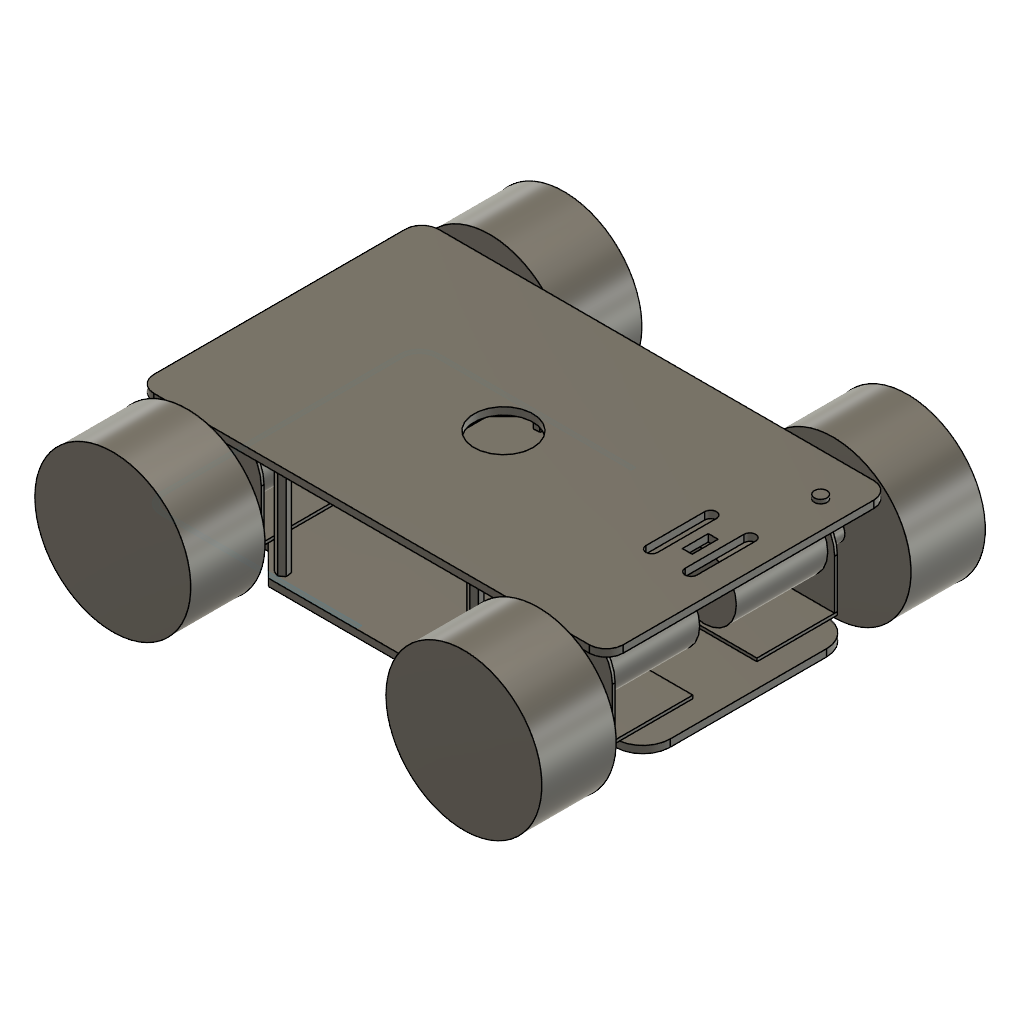
chassi migo base (Autodesk Fusion 360 design; units mm, degrees)
Autodesk Fusion 360 part; units mm, degrees
sketch "Esboço1" plane through (0, 0, 0) normal (0, 1, 0) x (1, 0, 0)
  line L0 (0, 0) -> (0, -111.6)
  line L1 (0, -111.6) -> (50, -111.6)
  line L2 (50, -111.6) -> (65.6125, -127.1)
  line L3 (65.6125, -127.1) -> (165.6125, -127.1)
  line L4 (165.6125, -127.1) -> (178.9919, -109.636)
  line L5 (178.9919, -109.636) -> (238.9919, -109.636)
  line L6 (238.9919, -109.636) -> (238.9919, -1.964)
  line L7 (238.9919, -1.964) -> (178.9919, -1.964)
  line L8 (178.9919, -1.964) -> (165.6125, 15.5)
  line L9 (165.6125, 15.5) -> (65.6125, 15.5)
  line L10 (65.6125, 15.5) -> (50, 0)
  line L11 (50, 0) -> (0, 0)
  dimension "d1" = 111.6
  dimension "d2" = 15.5
  dimension "d3" = 100
  dimension "d5" = 239
  dimension "d10" = 100
  dimension "d15" = 50
  dimension "d17" = 22
  dimension "d18" = 50
  dimension "d20" = 22
  dimension "d21" = 22
  dimension "d23" = 60
  dimension "d24" = 22
  dimension "d25" = 15.5
  dimension "d26" = 60
  constraint coincident L0.start L11.end
  constraint vertical L0
  constraint perpendicular L0 L1
  constraint perpendicular L0 L3
  constraint parallel L3 L5
  constraint perpendicular L5 L6
  constraint perpendicular L6 L7
  constraint perpendicular L6 L9
  constraint perpendicular L0 L11
  measures "d1" distance of L0.start L0.end
  measures "d2" distance of L1 L3
  measures "d3" distance of L2.end L3.end
  measures "d5" distance of L0.end L5.end
  measures "d10" distance of L8.end L9.end
  measures "d15" distance of L0.end L1.end
  measures "d17" distance of L1.end L2.end
  measures "d18" distance of L0.start L10.end
  measures "d20" distance of L7.end L8.end
  measures "d21" distance of L9.end L10.end
  measures "d23" distance of L6.end L7.end
  measures "d24" distance of L3.end L4.end
  measures "d25" vertical distance of L0.start L9.end
  measures "d26" distance of L4.end L5.end
extrude "Extrusão1" add sketch "Esboço1" along normal blind 3.7 makes body 1
fillet "Arredondamento1" radius 10 1 edges at (0, 1.85, 111.6) on bodies 1
fillet "Arredondamento2" radius 10 1 edges at (0, 1.85, 0) on bodies 1
fillet "Arredondamento3" radius 14 1 edges at (238.9919, 1.85, 109.636) on bodies 1
fillet "Arredondamento4" radius 14 1 edges at (238.9919, 1.85, 1.964) on bodies 1
sketch "Esboço2" plane through (0, 3.7, 0) normal (0, 1, 0) x (-1, 0, 0)
  arc A0 (-238.9919, 15.964) -> (-224.9919, 1.964) centre (-224.9919, 15.964) ccw
  line L0 (-224.9919, 1.964) -> (-178.9919, 1.964)
  line L1 (-178.9919, 1.964) -> (-165.6125, -15.5)
  line L2 (-165.6125, -15.5) -> (-65.6125, -15.5)
  line L3 (-65.6125, -15.5) -> (-50, 0)
  line L4 (-50, 0) -> (-10, 0)
  arc A1 (-10, 0) -> (0, 10) centre (-10, 10) ccw
  line L5 (0, 10) -> (0, 101.6)
  arc A2 (0, 101.6) -> (-10, 111.6) centre (-10, 101.6) ccw
  line L6 (-10, 111.6) -> (-50, 111.6)
  line L7 (-50, 111.6) -> (-65.6125, 127.1)
  line L8 (-65.6125, 127.1) -> (-165.6125, 127.1)
  line L9 (-165.6125, 127.1) -> (-178.9919, 109.636)
  line L10 (-178.9919, 109.636) -> (-224.9919, 109.636)
  arc A3 (-224.9919, 109.636) -> (-238.9919, 95.636) centre (-224.9919, 95.636) ccw
  line L11 (-238.9919, 95.636) -> (-238.9919, 15.964)
  line L12 (-69.4965, 121.884) -> (-69.0799, 118.7943)
  line L13 (-69.0799, 118.7943) -> (-66.1958, 117.6103)
  line L14 (-66.1958, 117.6103) -> (-63.7283, 119.516)
  line L15 (-63.7283, 119.516) -> (-64.145, 122.6057)
  line L16 (-64.145, 122.6057) -> (-67.0291, 123.7897)
  line L17 (-67.0291, 123.7897) -> (-69.4965, 121.884)
  line L18 (-167.5652, 122.0119) -> (-167.2872, 118.9067)
  line L19 (-167.2872, 118.9067) -> (-164.459, 117.5947)
  line L20 (-164.459, 117.5947) -> (-161.9087, 119.3881)
  line L21 (-161.9087, 119.3881) -> (-162.1867, 122.4933)
  line L22 (-162.1867, 122.4933) -> (-165.0149, 123.8053)
  line L23 (-165.0149, 123.8053) -> (-167.5652, 122.0119)
  line L24 (-70.3397, -6.4973) -> (-71.7356, -9.2851)
  line L25 (-71.7356, -9.2851) -> (-70.0192, -11.8878)
  line L26 (-70.0192, -11.8878) -> (-66.907, -11.7027)
  line L27 (-66.907, -11.7027) -> (-65.5112, -8.9149)
  line L28 (-65.5112, -8.9149) -> (-67.2275, -6.3122)
  line L29 (-67.2275, -6.3122) -> (-70.3397, -6.4973)
  line L30 (-167.9928, -8.5248) -> (-166.9588, -11.4661)
  line L31 (-166.9588, -11.4661) -> (-163.8946, -12.0412)
  line L32 (-163.8946, -12.0412) -> (-161.8644, -9.6752)
  line L33 (-161.8644, -9.6752) -> (-162.8984, -6.7339)
  line L34 (-162.8984, -6.7339) -> (-165.9625, -6.1588)
  line L35 (-165.9625, -6.1588) -> (-167.9928, -8.5248)
  point P0 (-66.6124, 120.7)
  point P1 (-164.7369, 120.7)
  point P2 (-68.6234, -9.1)
  point P3 (-164.9286, -9.1)
  dimension "d37" = 2.7
  dimension "d38" = 2.7
  dimension "d39" = 2.7
  dimension "d40" = 2.7
  dimension "d41" = 6.4
  dimension "d42" = 6.4
  dimension "d43" = 6.4
  dimension "d44" = 6.4
  measures "d37" distance of P0 L17
  measures "d38" distance of P1 L23
  measures "d39" distance of P2 L29
  measures "d40" distance of P3 L35
  measures "d41" distance of L8 P0
  measures "d42" distance of L8 P1
  measures "d43" distance of L2 P3
  measures "d44" distance of L2 P2
extrude "Extrusão2" add sketch "Esboço2" along normal blind 50 contours L12 L13 L14 L15 L16 L17 | L18 L19 L20 L21 L22 L23 | L24 L25 L26 L27 L28 L29 | L30 L31 L32 L33 L34 L35 bodies 1
sketch "Esboço3" plane through (0, 3.7, 0) normal (0, 1, 0) x (-1, 0, 0)
  line L0 (-67.2275, -6.3122) -> (-65.5112, -8.9149)
  line L1 (-65.5112, -8.9149) -> (-66.907, -11.7027)
  line L2 (-66.907, -11.7027) -> (-70.0192, -11.8878)
  line L3 (-70.0192, -11.8878) -> (-71.7356, -9.2851)
  line L4 (-71.7356, -9.2851) -> (-70.3397, -6.4973)
  line L5 (-70.3397, -6.4973) -> (-67.2275, -6.3122)
  line L6 (-67.0291, 123.7897) -> (-64.145, 122.6057)
  line L7 (-64.145, 122.6057) -> (-63.7283, 119.516)
  line L8 (-63.7283, 119.516) -> (-66.1958, 117.6103)
  line L9 (-66.1958, 117.6103) -> (-69.0799, 118.7943)
  line L10 (-69.0799, 118.7943) -> (-69.4965, 121.884)
  line L11 (-69.4965, 121.884) -> (-67.0291, 123.7897)
  line L12 (-165.9625, -6.1588) -> (-162.8984, -6.7339)
  line L13 (-162.8984, -6.7339) -> (-161.8644, -9.6752)
  line L14 (-161.8644, -9.6752) -> (-163.8946, -12.0412)
  line L15 (-163.8946, -12.0412) -> (-166.9588, -11.4661)
  line L16 (-166.9588, -11.4661) -> (-167.9928, -8.5248)
  line L17 (-167.9928, -8.5248) -> (-165.9625, -6.1588)
  line L18 (-165.0149, 123.8053) -> (-162.1867, 122.4933)
  line L19 (-162.1867, 122.4933) -> (-161.9087, 119.3881)
  line L20 (-161.9087, 119.3881) -> (-164.459, 117.5947)
  line L21 (-164.459, 117.5947) -> (-167.2872, 118.9067)
  line L22 (-167.2872, 118.9067) -> (-167.5652, 122.0119)
  line L23 (-167.5652, 122.0119) -> (-165.0149, 123.8053)
  arc A0 (-238.9919, 15.964) -> (-224.9919, 1.964) centre (-224.9919, 15.964) ccw
  line L24 (-224.9919, 1.964) -> (-178.9919, 1.964)
  line L25 (-178.9919, 1.964) -> (-165.6125, -15.5)
  line L26 (-165.6125, -15.5) -> (-65.6125, -15.5)
  line L27 (-65.6125, -15.5) -> (-50, 0)
  line L28 (-50, 0) -> (-10, 0)
  arc A1 (-10, 0) -> (0, 10) centre (-10, 10) ccw
  line L29 (0, 10) -> (0, 101.6)
  arc A2 (0, 101.6) -> (-10, 111.6) centre (-10, 101.6) ccw
  line L30 (-10, 111.6) -> (-50, 111.6)
  line L31 (-50, 111.6) -> (-65.6125, 127.1)
  line L32 (-65.6125, 127.1) -> (-165.6125, 127.1)
  line L33 (-165.6125, 127.1) -> (-178.9919, 109.636)
  line L34 (-178.9919, 109.636) -> (-224.9919, 109.636)
  arc A3 (-224.9919, 109.636) -> (-238.9919, 95.636) centre (-224.9919, 95.636) ccw
  line L35 (-238.9919, 95.636) -> (-238.9919, 15.964)
sketch "Esboço4" plane through (0, 3.7, 0) normal (0, 1, 0) x (-1, 0, 0)
  line L0 (-10, 74.1) -> (-50, 74.1)
  line L1 (-50, 74.1) -> (-50, 115.1)
  line L2 (-50, 115.1) -> (-10, 115.1)
  line L3 (-10, 115.1) -> (-10, 74.1)
  line L4 (0, 10) -> (0, 101.6)
  line L5 (-10, 111.6) -> (-50, 111.6)
  dimension "d47" = 10
  dimension "d48" = 40
  dimension "d49" = 41
  dimension "d50" = 3.5
  constraint horizontal L0
  constraint vertical L1
  constraint horizontal L2
  constraint vertical L3
  measures "d47" distance of L3 L4
  measures "d48" distance of L1.end L2.end
  measures "d49" distance of L0.end L1.end
  measures "d50" distance of L2 L5
sketch "Esboço5" plane through (0, 3.7, 0) normal (0, 1, 0) x (-1, 0, 0)
  line L0 (-186.9919, 72.136) -> (-226.9919, 72.136)
  line L1 (-226.9919, 72.136) -> (-226.9919, 113.136)
  line L2 (-226.9919, 113.136) -> (-186.9919, 113.136)
  line L3 (-186.9919, 113.136) -> (-186.9919, 72.136)
  line L4 (-238.9919, 95.636) -> (-238.9919, 15.964)
  line L5 (-178.9919, 109.636) -> (-224.9919, 109.636)
  dimension "d51" = 12
  dimension "d52" = 40
  dimension "d53" = 41
  dimension "d54" = 3.5
  constraint horizontal L0
  constraint vertical L1
  constraint horizontal L2
  constraint vertical L3
  measures "d51" distance of L1 L4
  measures "d52" distance of L0.start L0.end
  measures "d53" distance of L0.start L2.end
  measures "d54" distance of L2 L5
sketch "Esboço6" plane through (0, 3.7, 0) normal (0, 1, 0) x (-1, 0, 0)
  line L0 (-10, -3.5) -> (-50, -3.5)
  line L1 (-50, -3.5) -> (-50, 37.5)
  line L2 (-50, 37.5) -> (-10, 37.5)
  line L3 (-10, 37.5) -> (-10, -3.5)
  line L4 (-186.9919, -1.536) -> (-226.9919, -1.536)
  line L5 (-226.9919, -1.536) -> (-226.9919, 39.464)
  line L6 (-226.9919, 39.464) -> (-186.9919, 39.464)
  line L7 (-186.9919, 39.464) -> (-186.9919, -1.536)
  line L8 (-238.9919, 95.636) -> (-238.9919, 15.964)
  line L9 (-224.9919, 1.964) -> (-178.9919, 1.964)
  line L10 (0, 10) -> (0, 101.6)
  line L11 (-50, 0) -> (-10, 0)
  dimension "d55" = 40
  dimension "d56" = 41
  dimension "d57" = 40
  dimension "d58" = 41
  dimension "d59" = 12
  dimension "d61" = 3.5
  dimension "d62" = 10
  dimension "d63" = 3.5
  constraint horizontal L0
  constraint vertical L1
  constraint horizontal L2
  constraint vertical L3
  constraint horizontal L4
  constraint vertical L5
  constraint horizontal L6
  constraint vertical L7
  measures "d55" distance of L0.start L0.end
  measures "d56" distance of L0.start L2.end
  measures "d57" distance of L4.start L4.end
  measures "d58" distance of L4.start L6.end
  measures "d59" distance of L5 L8
  measures "d61" distance of L4 L9
  measures "d62" distance of L3 L10
  measures "d63" distance of L0 L11
extrude "Extrusão3" add sketch "Esboço6" sketch "Esboço4" sketch "Esboço5" along normal blind 1.6 of sketch 2 of sketch 3 bodies 1
sketch "Esboço7" plane through (0, 5.3, 0) normal (0, 1, 0) x (-1, 0, 0)
  line L0 (-10, 115.1) -> (-50, 115.1)
  line L1 (-50, 115.1) -> (-50, 74.1)
  line L2 (-50, 74.1) -> (-10, 74.1)
  line L3 (-10, 74.1) -> (-10, 115.1)
  line L4 (-10, 113.7) -> (-10, 115.1)
  line L5 (-10, 115.1) -> (-50, 115.1)
  line L6 (-50, 115.1) -> (-50, 113.7)
  line L7 (-50, 113.7) -> (-10, 113.7)
  dimension "d66" = 1.4
  constraint coincident L3 L4.start
  constraint coincident L0.start L3.end
  constraint coincident L0.end L1.start
  constraint coincident L1 L6.end
  constraint perpendicular L3 L7
  measures "d66" distance of L4.start L0.start
extrude "Extrusão4" add sketch "Esboço7" along normal blind 45.2 contours L0 L1 L3 L4 L5 L6 L7 bodies 1
sketch "Esboço8" plane through (0, 3.7, 0) normal (0, 1, 0) x (-1, 0, 0)
  line L0 (-0.1486, -16.5845) -> (-239.1486, -16.5845)
  line L1 (-239.1486, -16.5845) -> (-239.1486, 128.4155)
  line L2 (-239.1486, 128.4155) -> (-0.1486, 128.4155)
  line L3 (-0.1486, 128.4155) -> (-0.1486, -16.5845)
  line L4 (-238.9919, 95.636) -> (-238.9919, 15.964)
  dimension "d69" = 239
  dimension "d70" = 145
  constraint horizontal L0
  constraint vertical L1
  constraint horizontal L2
  constraint vertical L3
  measures "d69" distance of L0.start L0.end
  measures "d70" distance of L0.start L2.end
extrude "Extrusão5" add sketch "Esboço8" along normal blind 3.7 from surface at 50 bodies 1
fillet "Arredondamento5" radius 8.6 1 edges at (239.1486, 55.55, -16.5845) on bodies 1
fillet "Arredondamento6" radius 8.6 1 edges at (239.1486, 55.55, 128.4155) on bodies 1
fillet "Arredondamento7" radius 8.4 1 edges at (0.1486, 55.55, -16.5845) on bodies 1
fillet "Arredondamento8" radius 8.4 1 edges at (0.1486, 55.55, 128.4155) on bodies 1
fillet "Arredondamento9" radius 20 1 edges at (10, 50.5, 114.4) on bodies 1
fillet "Arredondamento10" radius 20 1 edges at (50, 50.5, 114.4) on bodies 1
sketch "Esboço9" plane through (0, 0, 115.1) normal (0, 0, 1) x (1, 0, 0)
  arc A0 (50, 30.5) -> (10, 30.5) centre (30, 30.5) ccw
  line L0 (10, 30.5) -> (10, 3.7)
  line L1 (10, 3.7) -> (50, 3.7)
  line L2 (50, 3.7) -> (50, 30.5)
  circle A1 centre (30, 23.7) radius 5.9
  dimension "d87" = 20
  dimension "d88" = 11.8
  measures "d87" distance of L1 A1.centre
  measures "d88" diameter of A1
extrude "Extrusão6" add sketch "Esboço9" along normal blind 5.8 contours A1 bodies 1
sketch "Esboço10" plane through (0, 0, 120.9) normal (0, 0, 1) x (1, 0, 0)
  circle A0 centre (30, 23.7) radius 5.9
  circle A1 centre (30, 23.7) radius 2.9
  dimension "d91" = 5.8
  constraint concentric A0 A1
  measures "d91" diameter of A1
extrude "Extrusão7" add sketch "Esboço10" along normal blind 15.4 contours A1 bodies 1
sketch "Esboço11" plane through (0, 0, 113.7) normal (0, 0, -1) x (-1, 0, 0)
  arc A0 (-10, 30.5) -> (-50, 30.5) centre (-30, 30.5) ccw
  line L0 (-50, 30.5) -> (-50, 5.3)
  line L1 (-50, 5.3) -> (-10, 5.3)
  line L2 (-10, 5.3) -> (-10, 30.5)
  circle A1 centre (-30, 30.5) radius 16.5
  dimension "d94" = 33
  constraint coincident A0.centre A1.centre
  measures "d94" diameter of A1
extrude "Extrusão8" add sketch "Esboço11" along normal blind 46.6 contours A1 bodies 1
sketch "Esboço12" plane through (0, 0, 0) normal (0, 0, 1) x (1, 0, 0)
  line L0 (10, 5.3) -> (50, 5.3)
  line L1 (50, 5.3) -> (50, 30.5)
  arc A0 (50, 30.5) -> (10, 30.5) centre (30, 30.5) ccw
  line L2 (10, 30.5) -> (10, 5.3)
extrude "Extrusão9" add sketch "Esboço12" along normal blind 1.4 from surface at -3.5 bodies 1
sketch "Esboço13" plane through (0, 0, 0) normal (0, 0, 1) x (1, 0, 0)
  circle A0 centre (30, 30.5) radius 16.5
extrude "Extrusão10" add sketch "Esboço13" along normal blind 46.6 from surface at -2.1 bodies 1
sketch "Esboço14" plane through (0, 0, 0) normal (0, 0, 1) x (1, 0, 0)
  circle A0 centre (30, 23.7) radius 5.9
extrude "Extrusão11" add sketch "Esboço14" along normal blind 5.8 from surface at -9.3 bodies 1
sketch "Esboço15" plane through (0, 0, 0) normal (0, 0, 1) x (1, 0, 0)
  circle A0 centre (30, 23.7) radius 2.9
extrude "Extrusão12" add sketch "Esboço15" along normal blind 15.4 from surface at -24.7 bodies 1
sketch "Esboço16" plane through (0, 0, 0) normal (0, 0, 1) x (1, 0, 0)
  line L0 (186.99, 5.3) -> (226.99, 5.3)
  line L1 (226.99, 5.3) -> (226.99, 30.5)
  arc A0 (226.99, 30.5) -> (186.99, 30.5) centre (206.99, 30.5) ccw
  line L2 (186.99, 30.5) -> (186.99, 5.3)
extrude "Extrusão13" add sketch "Esboço16" along normal blind 1.4 from surface at -1.54 bodies 1
sketch "Esboço17" plane through (0, 0, 0) normal (0, 0, 1) x (1, 0, 0)
  circle A0 centre (206.99, 30.5) radius 16.5
extrude "Extrusão14" add sketch "Esboço17" along normal blind 46.6 from surface at -0.14 bodies 1
sketch "Esboço18" plane through (0, 0, 0) normal (0, 0, 1) x (1, 0, 0)
  circle A0 centre (206.99, 23.7) radius 5.9
extrude "Extrusão15" add sketch "Esboço18" along normal blind 5.8 from surface at -7.34 bodies 1
sketch "Esboço19" plane through (0, 0, 0) normal (0, 0, 1) x (1, 0, 0)
  circle A0 centre (206.99, 23.7) radius 2.9
extrude "Extrusão16" add sketch "Esboço19" along normal blind 15.4 from surface at -22.74 bodies 1
sketch "Esboço20" plane through (0, 0, 0) normal (0, 0, 1) x (1, 0, 0)
  line L0 (186.99, 5.3) -> (226.99, 5.3)
  line L1 (226.99, 5.3) -> (226.99, 30.5)
  arc A0 (226.99, 30.5) -> (186.99, 30.5) centre (206.99, 30.5) ccw
  line L2 (186.99, 30.5) -> (186.99, 5.3)
extrude "Extrusão17" add sketch "Esboço20" along normal blind 1.4 from surface at 111.74 bodies 1
sketch "Esboço21" plane through (0, 0, 0) normal (0, 0, 1) x (1, 0, 0)
  circle A0 centre (206.99, 30.5) radius 16.5
extrude "Extrusão18" add sketch "Esboço21" along normal blind 46.6 from surface at 65.14 bodies 1
sketch "Esboço22" plane through (0, 0, 0) normal (0, 0, 1) x (1, 0, 0)
  circle A0 centre (206.99, 23.7) radius 5.9
extrude "Extrusão19" add sketch "Esboço22" along normal blind 5.8 from surface at 113.14 bodies 1
sketch "Esboço23" plane through (0, 0, 0) normal (0, 0, 1) x (1, 0, 0)
  circle A0 centre (206.99, 23.7) radius 2.9
extrude "Extrusão20" add sketch "Esboço23" along normal blind 15.4 from surface at 118.94 bodies 1
sketch "Esboço24" plane through (0, 57.4, 0) normal (0, 1, 0) x (-1, 0, 0)
  arc A0 (-0.1486, 120.0155) -> (-8.5486, 128.4155) centre (-8.5486, 120.0155) ccw
  line L0 (-8.5486, 128.4155) -> (-230.5486, 128.4155)
  arc A1 (-230.5486, 128.4155) -> (-239.1486, 119.8155) centre (-230.5486, 119.8155) ccw
  line L1 (-239.1486, 119.8155) -> (-239.1486, -7.9845)
  arc A2 (-239.1486, -7.9845) -> (-230.5486, -16.5845) centre (-230.5486, -7.9845) ccw
  line L2 (-230.5486, -16.5845) -> (-8.5486, -16.5845)
  arc A3 (-8.5486, -16.5845) -> (-0.1486, -8.1845) centre (-8.5486, -8.1845) ccw
  line L3 (-0.1486, -8.1845) -> (-0.1486, 120.0155)
sketch "Esboço25" plane through (0, 57.4, 0) normal (0, 1, 0) x (-1, 0, 0)
  circle A0 centre (-225, 5) radius 3.2443
extrude "Extrusão21" add sketch "Esboço25" along normal blind 2 bodies 1
sketch "Esboço26" plane through (0, 57.4, 0) normal (0, 1, 0) x (-1, 0, 0)
  circle A0 centre (-114.1486, 55.8) radius 15
  line L0 (-239.1486, 119.8155) -> (-239.1486, -7.9845)
  line L1 (-8.5486, 128.4155) -> (-230.5486, 128.4155)
  line L2 (-65.6125, 127.1) -> (-165.6125, 127.1)
  dimension "d135" = 30
  dimension "d136" = 125
  dimension "d139" = 71.3
  measures "d135" diameter of A0
  measures "d136" distance of A0.centre L0
  measures "d139" distance of A0.centre L2
extrude "Extrusão22" cut sketch "Esboço26" against normal blind 4 bodies 1
sketch "Esboço27" plane through (0, 57.4, 0) normal (0, 1, 0) x (-1, 0, 0)
  line L0 (-227.1486, 73.2155) -> (-221.1486, 73.2155)
  line L1 (-221.1486, 73.2155) -> (-221.1486, 37.2155)
  line L2 (-221.1486, 37.2155) -> (-227.1486, 37.2155)
  line L3 (-227.1486, 37.2155) -> (-227.1486, 73.2155)
  line L4 (-207.1486, 73.2155) -> (-201.1486, 73.2155)
  line L5 (-201.1486, 73.2155) -> (-201.1486, 37.2155)
  line L6 (-201.1486, 37.2155) -> (-207.1486, 37.2155)
  line L7 (-207.1486, 37.2155) -> (-207.1486, 73.2155)
  line L8 (-216.7486, 62.2155) -> (-211.7486, 62.2155)
  line L9 (-211.7486, 62.2155) -> (-211.7486, 49.0155)
  line L10 (-211.7486, 49.0155) -> (-216.7486, 49.0155)
  line L11 (-216.7486, 49.0155) -> (-216.7486, 62.2155)
  line L12 (-239.1486, 119.8155) -> (-239.1486, -7.9845)
  line L13 (-8.5486, 128.4155) -> (-230.5486, 128.4155)
  dimension "d142" = 6
  dimension "d143" = 36
  dimension "d144" = 6
  dimension "d145" = 36
  dimension "d146" = 5
  dimension "d147" = 13.2
  dimension "d148" = 12
  dimension "d149" = 55.2
  dimension "d150" = 55.2
  dimension "d151" = 66.2
  dimension "d152" = 32
  dimension "d153" = 22.4
  constraint horizontal L0
  constraint vertical L1
  constraint horizontal L2
  constraint vertical L3
  constraint horizontal L4
  constraint vertical L5
  constraint horizontal L6
  constraint vertical L7
  constraint horizontal L8
  constraint vertical L9
  constraint horizontal L10
  constraint vertical L11
  measures "d142" distance of L0.start L0.end
  measures "d143" distance of L0.start L2.end
  measures "d144" distance of L4.start L4.end
  measures "d145" distance of L4.start L6.end
  measures "d146" distance of L8.start L8.end
  measures "d147" distance of L8.start L10.end
  measures "d148" distance of L3 L12
  measures "d149" distance of L0 L13
  measures "d150" distance of L4 L13
  measures "d151" distance of L8 L13
  measures "d152" distance of L7 L12
  measures "d153" distance of L11 L12
extrude "Extrusão23" cut sketch "Esboço27" against normal blind 4 bodies 1
fillet "Arredondamento11" radius 3 4 edges at (221.1486, 55.55, 73.2155) (227.1486, 55.55, 73.2155) (221.1486, 55.55, 37.2155) (227.1486, 55.55, 37.2155) on bodies 1
fillet "Arredondamento12" radius 3 4 edges at (207.1486, 55.55, 37.2155) (201.1486, 55.55, 37.2155) (201.1486, 55.55, 73.2155) (207.1486, 55.55, 73.2155) on bodies 1
sketch "Esboço28" plane through (0, 0, 0) normal (0, 0, 1) x (1, 0, 0)
  circle A0 centre (30, 23.7) radius 40
sketch "Esboço29" plane through (0, 0, 0) normal (0, 0, 1) x (1, 0, 0)
  circle A0 centre (206.99, 23.7) radius 40
sketch "Esboço30" plane through (0, 0, 0) normal (0, 0, 1) x (1, 0, 0)
  circle A0 centre (206.99, 23.7) radius 40
sketch "Esboço31" plane through (0, 0, 0) normal (0, 0, 1) x (1, 0, 0)
  circle A0 centre (30, 23.7) radius 40
sketch "Esboço32" plane through (0, 0, 0) normal (0, 0, 1) x (1, 0, 0)
  circle A0 centre (30, 23.7) radius 6
sketch "Esboço33" plane through (0, 0, 0) normal (0, 0, 1) x (1, 0, 0)
  circle A0 centre (30, 23.7) radius 39.75
sketch "Esboço34" plane through (0, 0, 0) normal (0, 0, 1) x (1, 0, 0)
  circle A0 centre (206.99, 23.7) radius 6
sketch "Esboço35" plane through (0, 0, 0) normal (0, 0, 1) x (1, 0, 0)
  circle A0 centre (206.99, 23.7) radius 39.75
sketch "Esboço36" plane through (0, 0, 0) normal (0, 0, 1) x (1, 0, 0)
  circle A0 centre (206.99, 23.7) radius 6
sketch "Esboço37" plane through (0, 0, 0) normal (0, 0, 1) x (1, 0, 0)
  circle A0 centre (206.99, 23.7) radius 39.75
sketch "Esboço38" plane through (0, 0, 0) normal (0, 0, 1) x (1, 0, 0)
  circle A0 centre (30, 23.7) radius 6
sketch "Esboço39" plane through (0, 0, 0) normal (0, 0, 1) x (1, 0, 0)
  circle A0 centre (30, 23.7) radius 39.75
sketch "Esboço40" plane through (0, 0, 0) normal (0, 0, 1) x (1, 0, 0)
  circle A0 centre (30, 23.7) radius 6
extrude "Extrusão36" add sketch "Esboço40" along normal blind 12 from surface at -21.3 separate body makes body 2
sketch "Esboço41" plane through (0, 0, 0) normal (0, 0, 1) x (1, 0, 0)
  circle A0 centre (30, 23.7) radius 39.75
extrude "Extrusão37" add sketch "Esboço41" along normal blind 37.9 from surface at -59.2 separate body makes body 3
sketch "Esboço42" plane through (0, 0, 0) normal (0, 0, 1) x (1, 0, 0)
  circle A0 centre (206.99, 23.7) radius 6
extrude "Extrusão38" add sketch "Esboço42" along normal blind 12 from surface at -19.34 separate body makes body 4
sketch "Esboço43" plane through (0, 0, 0) normal (0, 0, 1) x (1, 0, 0)
  circle A0 centre (206.99, 23.7) radius 39.75
extrude "Extrusão39" add sketch "Esboço43" along normal blind 37.9 from surface at -57.24 separate body makes body 5
sketch "Esboço44" plane through (0, 0, 0) normal (0, 0, 1) x (1, 0, 0)
  circle A0 centre (206.99, 23.7) radius 6
extrude "Extrusão40" add sketch "Esboço44" along normal blind 12 from surface at 118.94 separate body makes body 6
sketch "Esboço45" plane through (0, 0, 0) normal (0, 0, 1) x (1, 0, 0)
  circle A0 centre (206.99, 23.7) radius 39.75
extrude "Extrusão41" add sketch "Esboço45" along normal blind 37.9 from surface at 130.94 separate body makes body 7
sketch "Esboço46" plane through (0, 0, 0) normal (0, 0, 1) x (1, 0, 0)
  circle A0 centre (30, 23.7) radius 6
extrude "Extrusão42" add sketch "Esboço46" along normal blind 12 from surface at 120.9 separate body makes body 8
sketch "Esboço47" plane through (0, 0, 0) normal (0, 0, 1) x (1, 0, 0)
  circle A0 centre (30, 23.7) radius 39.75
extrude "Extrusão43" add sketch "Esboço47" along normal blind 37.9 from surface at 132.9 separate body makes body 9
sketch "Esboço48" plane through (0, 3.9, 0) normal (0, -1, 0) x (1, 0, 0)
  line L0 (110.5845, 124.4) -> (110.5845, 126.8)
  line L1 (110.5845, 126.8) -> (10.3, 126.8)
  arc A0 (10.3, 126.8) -> (0.3, 116.8) centre (10.3, 116.8) ccw
  line L2 (0.3, 116.8) -> (0.3, -5.2)
  arc A1 (0.3, -5.2) -> (10.3, -15.2) centre (10.3, -5.2) ccw
  line L3 (10.3, -15.2) -> (110.5845, -15.2)
  line L4 (110.5845, -15.2) -> (110.5845, -12.8)
  line L5 (110.5845, -12.8) -> (10.7, -12.8)
  arc A2 (2.7, -4.8) -> (10.7, -12.8) centre (10.7, -4.8) ccw
  line L6 (2.7, -4.8) -> (2.7, 116.4)
  arc A3 (10.7, 124.4) -> (2.7, 116.4) centre (10.7, 116.4) ccw
  line L7 (10.7, 124.4) -> (110.5845, 124.4)
named bodies: "acopl_A", "roda_A", "acopl_B", "roda_B", "acopl_C", "roda_C", "acopl_D", "roda_D"
